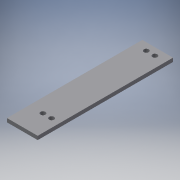
# Autodesk Inventor part: Ball screw rear-end support
Saved by Autodesk Inventor 2016 (Build 200138000, 138)
## iProperties
Created: 2017-07-25
Part Number: Ball screw rear-end support
Material: Generic
Document SubType Name: Modeling
Designer: m228540
Density: 1 g/cm^3
Appearance: Default
Author: m228540
Autodesk Inventor part; units mm, degrees
ref_plane "YZ Plane" through (0, 0, 0) normal (1, 0, 0) x (0, 1, 0)
ref_plane "XZ Plane" through (0, 0, 0) normal (0, 1, 0) x (-1, 0, 0)
ref_plane "XY Plane" through (0, 0, 0) normal (0, 0, 1) x (1, 0, 0)
sketch "Sketch1" plane through (0, 0, 0) normal (0, 0, 1) x (1, 0, 0)
  line L0 (-19.4215, 49.2769) -> (30.5785, 49.2769)
  line L1 (30.5785, 49.2769) -> (30.5785, -170.7231)
  line L2 (30.5785, -170.7231) -> (-19.4215, -170.7231)
  line L3 (-19.4215, -170.7231) -> (-19.4215, 49.2769)
  point P0 (0, 0)
  dimension "d0" = 50
  dimension "d1" = 220
  constraints: 8 end point, 2 parallel, 1 horizontal, 1 perpendicular
  measures "d0" distance of L0.start L0.end
  measures "d1" distance of L0.end L1.end
extrude "Extrusion1" add sketch "Sketch1" along normal mid plane 6
sketch "Sketch2" plane through (0, 0, -3) normal (0, 0, -1) x (-1, 0, 0)
  circle A0 centre (0.9215, 37.2769) radius 4 projected
  circle A1 centre (-13.0785, 37.2769) radius 4 projected
  circle A2 centre (-4.5785, -134.7231) radius 4 projected
  circle A3 centre (-18.5785, -134.7231) radius 4 projected
  point P0 (0, 0)
extrude "Extrusion2" cut sketch "Sketch2" against normal through all
sketch "Sketch3" plane through (0, 0, -3) normal (0, 0, -1) x (-1, 0, 0)
  circle A0 centre (-0.5785, 7.7769) radius 4.5 projected
  circle A1 centre (-0.5785, -52.2231) radius 4.5 projected
  point P0 (0, 0)
extrude "Extrusion3" cut sketch "Sketch3" against normal through all
body "Solid1"
